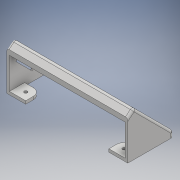
# Autodesk Inventor part: holder-LCD-screen
Saved by Autodesk Inventor 2018 (Build 220112000, 112)
## iProperties
Created: 2017-11-05
Part Number: holder-LCD-screen
Material: Generic
Document SubType Name: Modeling
Designer: Jurjen
Density: 1 g/cm^3
Appearance: Default
Author: Jurjen
Autodesk Inventor part; units mm, degrees
ref_plane "YZ Plane" through (0, 0, 0) normal (1, 0, 0) x (0, 1, 0)
ref_plane "XZ Plane" through (0, 0, 0) normal (0, 1, 0) x (-1, 0, 0)
ref_plane "XY Plane" through (0, 0, 0) normal (0, 0, 1) x (1, 0, 0)
sketch "Sketch1" plane through (0, 0, 0) normal (1, 0, 0) x (0, 1, 0)
  line L0 (-30, 25.7931) -> (-30, -25.7931)
  line L1 (30, -18.7931) -> (-21.6188, 32.8257)
  line L2 (-21.6188, 32.8257) -> (-30, 25.7931)
  line L3 (30, -18.7931) -> (30, -25.7931)
  line L4 (30, -25.7931) -> (-30, -25.7931)
  point P0 (0, 0)
  point P1 (-30, 0)
  point P2 (0, -25.7931)
  point P3 (-30, 0)
  dimension "d3" = 50
  dimension "d4" = 73
  dimension "d8" = 60
  dimension "d9" = 45
  dimension "d10" = 7
  constraints: 10 end point, 3 midpoint, 2 horizontal alignment, 2 vertical, 1 perpendicular, 1 vertical alignment
  measures "d3" angle of L2 L0
  measures "d4" distance of L1.start L1.end
  measures "d8" distance of L3.end L0.end
  measures "d9" angle of L4 L1
  measures "d10" distance of L1.start L3.end
extrude "Extrusion1" add sketch "Sketch1" along normal mid plane 160
sketch "Sketch2" plane through (-80, -21.6188, 32.8257) normal (0, 0.7071068, 0.7071068) x (1, 0, 0)
  line L0 (3.5, 69.5) -> (156.5, 69.5)
  line L1 (156.5, 69.5) -> (156.5, 3.5)
  line L2 (156.5, 3.5) -> (3.5, 3.5)
  line L3 (3.5, 3.5) -> (3.5, 69.5)
  line L4 (0, 0) -> (0, 73) projected
  line L5 (0, 0) -> (160, 0) projected
  line L6 (0, 73) -> (160, 73) projected
  line L7 (160, 73) -> (160, 0) projected
  point P0 (80, 38.4981)
  dimension "d11" = 3.5
  dimension "d12" = 3.5
  dimension "d13" = 3.5
  dimension "d14" = 3.5
  constraints: 8 end point, 2 parallel, 1 horizontal, 1 perpendicular
  measures "d11" distance between parallel lines of L4 L3
  measures "d12" distance between parallel lines of L5 L2
  measures "d13" distance between parallel lines of L6 L0
  measures "d14" distance between parallel lines of L7 L1
extrude "Extrusion2" cut sketch "Sketch2" against normal up to next contours L0 L1 L2 L3
sketch "Sketch3" plane through (-80, -21.6188, 32.8257) normal (0, 0.7071068, 0.7071068) x (1, 0, 0)
  line L0 (3.5, 3.5) -> (3.5, 69.5) projected
  line L1 (3.5, 69.5) -> (156.5, 69.5) projected
  line L2 (156.5, 69.5) -> (156.5, 3.5) projected
  line L3 (156.5, 3.5) -> (3.5, 3.5) projected
  line L4 (0, 0) -> (160, 0) projected
  line L5 (160, 73) -> (160, 0) projected
  line L6 (0, 73) -> (160, 73) projected
  line L7 (0, 0) -> (0, 73) projected
  line L8 (3.5, 69.5) -> (156.5, 69.5)
  line L9 (156.5, 69.5) -> (156.5, 3.5)
  line L10 (156.5, 3.5) -> (3.5, 3.5)
  line L11 (3.5, 3.5) -> (3.5, 69.5)
  line L12 (17.2, 55) -> (116.2, 55)
  line L13 (116.2, 55) -> (116.2, 14.5)
  line L14 (116.2, 14.5) -> (17.2, 14.5)
  line L15 (17.2, 14.5) -> (17.2, 55)
  circle A0 centre (142.6, 38.45) radius 2.75
  arc A1 (143.6, 56.45) -> (141.6, 56.45) centre (142.6, 56.45) ccw
  arc A2 (141.6, 52.45) -> (143.6, 52.45) centre (142.6, 52.45) ccw
  arc A3 (140.6, 54.95) -> (138.6, 54.95) centre (139.6, 54.95) ccw
  line L16 (141.6, 52.45) -> (141.6, 56.45)
  line L17 (143.6, 56.45) -> (143.6, 52.45)
  arc A4 (138.6, 53.95) -> (140.6, 53.95) centre (139.6, 53.95) ccw
  line L18 (138.6, 53.95) -> (138.6, 54.95)
  line L19 (140.6, 54.95) -> (140.6, 53.95)
  line L20 (142.6, 52.45) -> (142.6, 56.45) construction
  arc A5 (146.6, 54.95) -> (144.6, 54.95) centre (145.6, 54.95) ccw
  arc A6 (144.6, 53.95) -> (146.6, 53.95) centre (145.6, 53.95) ccw
  line L21 (146.6, 53.95) -> (146.6, 54.95)
  line L22 (144.6, 54.95) -> (144.6, 53.95)
  point P0 (80, 38.4981)
  dimension "d17" = 99
  dimension "d18" = 40.5
  dimension "d19" = 26.4
  dimension "d20" = 5.5
  dimension "d21" = 23.95
  dimension "d22" = 13.7
  dimension "d23" = 11
  dimension "d24" = 2
  dimension "d25" = 4
  dimension "d26" = 3
  dimension "d27" = 1.5
  dimension "d28" = 1.5
  dimension "d29" = 14
  constraints: 30 end point, 14 point on circle, 7 centre point, 7 symmetric about line, 6 tangent, 5 parallel, 3 equal radius, 3 vertical alignment, 2 horizontal, 2 perpendicular, 2 point on line, 2 vertical, 2 other
  measures "d17" distance between parallel lines of L13 L15
  measures "d18" distance between parallel lines of L14 L12
  measures "d19" distance from line of L13 A0.centre
  measures "d20" diameter of A0
  measures "d21" distance from line of A0.centre L14
  measures "d22" distance between parallel lines of L0 L15
  measures "d23" distance between parallel lines of L3 L14
  measures "d24" diameter of A1
  measures "d25" distance of L17.end L17.start
  measures "d26" horizontal distance of L20.end A3.centre
  measures "d27" vertical distance of L20.end A3.centre
  measures "d28" vertical distance of A4.centre L20.start
  measures "d29" distance of A0.centre L20.start
extrude "Extrusion3" add sketch "Sketch3" against normal blind 3 contours L0 L1 L2 L3
fillet "Fillet1" radius 3 8 edges at (0, -21.6188, 32.8257) (-80, 4.1906, 7.0163) (-80, -25.8094, 29.3094) (80, -25.8094, 29.3094) (80, 4.1906, 7.0163) (0, 30, -18.7931) (-80, 30, -22.2931) (80, 30, -22.2931)
sketch "Sketch4" plane through (76.5, 18.0503, -25.7931) normal (0, 0, -1) x (-1, 0, 0)
  line L0 (139.3, -2.8995) -> (139.3, -31.5373) projected
  line L1 (139.3, -31.5373) -> (40.3, -31.5373) projected
  line L2 (40.3, -31.5373) -> (40.3, -2.8995) projected
  line L3 (40.3, -2.8995) -> (139.3, -2.8995) projected
  ellipse E0 centre (13.9, -14.6021) end of major axis (16.65, -14.6021) minor radius 1.9445 projected
  line L4 (12.9, -4.7026) -> (12.9, -1.8742) projected
  ellipse E1 centre (13.9, -1.8742) end of major axis (12.9, -1.8742) minor radius 0.7071 (14.9, -1.8742) -> (12.9, -1.8742) ccw projected
  line L5 (14.9, -1.8742) -> (14.9, -4.7026) projected
  ellipse E2 centre (13.9, -4.7026) end of major axis (14.9, -4.7026) minor radius 0.7071 (12.9, -4.7026) -> (14.9, -4.7026) ccw projected
  ellipse E3 centre (10.9, -3.642) end of major axis (11.9, -3.642) minor radius 0.7071 (9.9, -3.642) -> (11.9, -3.642) ccw projected
  line L6 (9.9, -3.642) -> (9.9, -2.9349) projected
  ellipse E4 centre (10.9, -2.9349) end of major axis (9.9, -2.9349) minor radius 0.7071 (11.9, -2.9349) -> (9.9, -2.9349) ccw projected
  line L7 (11.9, -2.9349) -> (11.9, -3.642) projected
  ellipse E5 centre (16.9, -3.642) end of major axis (17.9, -3.642) minor radius 0.7071 (15.9, -3.642) -> (17.9, -3.642) ccw projected
  line L8 (15.9, -3.642) -> (15.9, -2.9349) projected
  ellipse E6 centre (16.9, -2.9349) end of major axis (15.9, -2.9349) minor radius 0.7071 (17.9, -2.9349) -> (15.9, -2.9349) ccw projected
  line L9 (17.9, -2.9349) -> (17.9, -3.642) projected
  line L10 (153, 7.3536) -> (153, -39.3155) projected
  line L11 (0, 7.3536) -> (153, 7.3536) projected
  line L12 (0, -39.3155) -> (0, 7.3536) projected
  line L13 (153, -39.3155) -> (0, -39.3155) projected
  line L14 (153, 0) -> (153, -48.0503) projected
  line L15 (0, 7.3536) -> (153, 7.3536)
  line L16 (153, 7.3536) -> (153, 0)
  line L17 (153, 0) -> (0, 0)
  line L18 (0, 0) -> (0, 7.3536)
  point P0 (76.5, -18.0503)
  constraints: 8 end point, 2 parallel, 1 horizontal, 1 perpendicular, 7 other
extrude "Extrusion4" cut sketch "Sketch4" against normal up to next contours L10 L17 L12 L11
sketch "Sketch5" plane through (-80, 0, 0) normal (-1, 0, 0) x (0, 0, 1)
  line L0 (-13.3123, -0.2295) -> (7.9009, -21.4427)
  line L1 (7.9009, -21.4427) -> (12.1436, -17.2001)
  line L2 (12.1436, -17.2001) -> (-9.0696, 4.0131)
  line L3 (-9.0696, 4.0131) -> (-13.3123, -0.2295)
  line L4 (-20.0357, 27) -> (28.7606, -21.7963) projected
  line L5 (28.2295, -21.2652) -> (-18.4395, 25.4038) projected
  line L6 (-18.4395, 25.4038) -> (28.2295, -21.2652) projected
  line L7 (-7.444, 14.4083) -> (-7.444, 14.4083) projected
  line L8 (-7.444, 14.4083) -> (-8.1511, 15.1154) projected
  line L9 (-8.1511, 15.1154) -> (-8.1511, 15.1154) projected
  line L10 (-8.1511, 15.1154) -> (-7.444, 14.4083) projected
  line L11 (-7.444, 14.4083) -> (-7.444, 14.4083) projected
  line L12 (-7.444, 14.4083) -> (-8.1511, 15.1154) projected
  line L13 (-8.1511, 15.1154) -> (-8.1511, 15.1154) projected
  line L14 (-8.1511, 15.1154) -> (-7.444, 14.4083) projected
  line L15 (-6.3833, 13.3476) -> (-9.2118, 16.1761) projected
  line L16 (-9.2118, 16.1761) -> (-9.2118, 16.1761) projected
  line L17 (-9.2118, 16.1761) -> (-6.3833, 13.3476) projected
  line L18 (-6.3833, 13.3476) -> (-6.3833, 13.3476) projected
  line L19 (5.4607, 1.5036) -> (1.5716, 5.3927) projected
  line L20 (-8.1865, 15.1508) -> (20.4514, -13.4871) projected
  line L21 (20.4514, -13.4871) -> (-8.1865, 15.1508) projected
  point P0 (0, 0)
  dimension "d35" = 30
  dimension "d36" = 6
  dimension "d39" = 14.5
  dimension "d40" = 15
  constraints: 8 end point, 3 perpendicular, 1 parallel
  measures "d35" distance of L1.end L2.end
  measures "d36" distance between parallel lines of L2 L0
  measures "d39" distance between parallel lines of L4 L0
  measures "d40" distance from line of L4.end L1
extrude "Extrusion5" cut sketch "Sketch5" against normal up to next
sketch "Sketch6" plane through (-77, -19.675, 30.8819) normal (0, 0.7071068, 0.7071068) x (1, 0, 0)
  circle A0 centre (4.1, 61.451) radius 1.6
  circle A1 centre (4.1, 11.951) radius 1.6
  circle A2 centre (148.6, 61.451) radius 1.6
  circle A3 centre (148.6, 11.951) radius 1.6
  line L0 (0.5, 71.9508) -> (0.5, 32.7743) projected
  line L1 (0.5, 0.751) -> (153.5, 0.751) projected
  point P0 (77, 35.7491)
  dimension "d41" = 3.2
  dimension "d42" = 144.5
  dimension "d43" = 49.5
  dimension "d44" = 3.6
  dimension "d45" = 11.2
  constraints: 4 centre point, 3 equal radius, 2 horizontal alignment, 2 vertical alignment
  measures "d41" diameter of A0
  measures "d42" distance of A2.centre A0.centre
  measures "d43" distance of A0.centre A1.centre
  measures "d44" distance from line of A0.centre L0
  measures "d45" distance from line of A1.centre L1
extrude "Extrusion6" cut sketch "Sketch6" against normal up to next
chamfer "Chamfer1" distance 2 angle 45 4 edges at (-80, -10.8361, -2.7057) (-80, 1.8918, -11.191) (-80, -6.5935, 1.537) (-80, -19.3214, 10.0222)
sketch "Sketch7" plane through (77, 30, -25.7931) normal (0, 0, -1) x (-1, 0, 0)
  line L0 (157, -51.7963) -> (157, -60) projected
  line L1 (157, -60) -> (132, -60)
  line L2 (132, -60) -> (132, -40)
  line L3 (132, -40) -> (157, -40)
  line L4 (157, -40) -> (157, -60)
  point P0 (77, -30)
  dimension "d51" = 25
  dimension "d52" = 20
  constraints: 8 end point, 2 parallel, 1 horizontal, 1 perpendicular
  measures "d51" distance between parallel lines of L4 L2
  measures "d52" distance between parallel lines of L1 L3
extrude "Extrusion7" add sketch "Sketch7" against normal blind 4
sketch "Sketch8" plane through (77, 30, -25.7931) normal (0, 0, -1) x (-1, 0, 0)
  circle A0 centre (142, -50) radius 2.1
  line L0 (157, -60) -> (132, -60) projected
  line L1 (132, -60) -> (132, -40) projected
  point P0 (77, -30)
  dimension "d55" = 10
  dimension "d56" = 10
  dimension "d57" = 4.2
  constraints: 1 centre point
  measures "d55" distance from line of L0 A0.centre
  measures "d56" distance from line of L1 A0.centre
  measures "d57" diameter of A0
fillet "Fillet2" radius 10 1 edges at (-55, -10, -23.7931)
extrude "Extrusion8" cut sketch "Sketch8" against normal up to next
mirror "Mirror1" about plane through (0, 0, 0) normal (1, 0, 0) of "Extrusion7", "Fillet2", "Extrusion8"
sketch "Sketch9" plane through (-77, -19.675, 30.8819) normal (0, 0.7071068, 0.7071068) x (1, 0, 0)
  line L0 (14.2, 64.6999) -> (52.5715, 64.6999) construction
  line L1 (52.5715, 64.6999) -> (52.5715, 56.5594) construction
  line L2 (52.5715, 56.5594) -> (14.2, 56.5594) construction
  line L3 (14.2, 56.5594) -> (14.2, 64.6999) construction
  line L4 (14.2, 52.251) -> (113.2, 52.251) projected
  line L5 (0, 69.0084) -> (154, 69.0084) projected
  line L6 (113.2, 52.251) -> (113.2, 69.0084) construction
  line L7 (20.0476, 60.6463) -> (18.5354, 60.3719)
  spline S0 degree 2 poles (18.5354, 60.3719) (18.4622, 60.8231) (17.9195, 61.2804) (17.4866, 61.2804) knots 0 0 0 1 2 2 2
  spline S1 degree 2 poles (17.4866, 61.2804) (16.9195, 61.2804) (16.2366, 60.4877) (16.2366, 59.5609) knots 0 0 0 1 2 2 2
  spline S2 degree 2 poles (16.2366, 59.5609) (16.2366, 58.5304) (16.9317, 57.6829) (17.511, 57.6829) knots 0 0 0 1 2 2 2
  spline S3 degree 2 poles (17.511, 57.6829) (17.95, 57.6829) (18.5049, 58.1829) (18.6207, 58.7865) knots 0 0 0 1 2 2 2
  line L8 (18.6207, 58.7865) -> (20.1268, 58.5304)
  spline S4 degree 2 poles (20.1268, 58.5304) (19.8951, 57.4938) (18.5598, 56.4329) (17.4439, 56.4329) knots 0 0 0 1 2 2 2
  spline S5 degree 2 poles (17.4439, 56.4329) (16.1756, 56.4329) (14.6634, 58.0365) (14.6634, 59.4572) knots 0 0 0 1 2 2 2
  spline S6 degree 2 poles (14.6634, 59.4572) (14.6634, 60.8902) (16.1756, 62.4877) (17.4683, 62.4877) knots 0 0 0 1 2 2 2
  spline S7 degree 2 poles (17.4683, 62.4877) (18.5293, 62.4877) (19.7732, 61.5792) (20.0476, 60.6463) knots 0 0 0 1 2 2 2
  spline S8 degree 2 poles (20.8585, 59.5426) (20.8585, 60.3048) (21.6146, 61.7377) (22.9927, 62.4877) (23.8463, 62.4877) knots 0 0 0 1 2 3 3 3
  spline S9 degree 2 poles (23.8463, 62.4877) (25.1634, 62.4877) (26.8463, 60.7804) (26.8463, 59.4755) knots 0 0 0 1 2 2 2
  spline S10 degree 2 poles (26.8463, 59.4755) (26.8463, 58.1646) (25.1451, 56.4329) (23.8585, 56.4329) knots 0 0 0 1 2 2 2
  spline S11 degree 2 poles (23.8585, 56.4329) (23.0598, 56.4329) (21.6146, 57.1524) (20.8585, 58.5426) (20.8585, 59.5426) knots 0 0 0 1 2 3 3 3
  spline S12 degree 2 poles (22.4317, 59.4633) (22.4317, 58.5975) (23.2488, 57.6829) (23.8524, 57.6829) knots 0 0 0 1 2 2 2
  spline S13 degree 2 poles (23.8524, 57.6829) (24.4561, 57.6829) (25.2671, 58.5975) (25.2671, 59.4694) knots 0 0 0 1 2 2 2
  spline S14 degree 2 poles (25.2671, 59.4694) (25.2671, 60.3231) (24.4561, 61.2377) (23.8524, 61.2377) knots 0 0 0 1 2 2 2
  spline S15 degree 2 poles (23.8524, 61.2377) (23.2488, 61.2377) (22.4317, 60.3231) (22.4317, 59.4633) knots 0 0 0 1 2 2 2
  line L9 (29.5171, 56.5609) -> (27.9805, 56.5609)
  line L10 (27.9805, 56.5609) -> (27.9805, 62.3597)
  line L11 (27.9805, 62.3597) -> (29.4073, 62.3597)
  line L12 (29.4073, 62.3597) -> (29.4073, 61.5365)
  spline S16 degree 2 poles (29.4073, 61.5365) (29.7732, 62.1219) (30.3524, 62.4877) (30.7244, 62.4877) knots 0 0 0 1 2 2 2
  spline S17 degree 2 poles (30.7244, 62.4877) (31.2488, 62.4877) (31.7305, 62.1951) knots 0 0 0 1 1 1
  line L13 (31.7305, 62.1951) -> (31.261, 60.8597)
  spline S18 degree 2 poles (31.261, 60.8597) (30.8707, 61.1097) (30.5415, 61.1097) knots 0 0 0 1 1 1
  spline S19 degree 2 poles (30.5415, 61.1097) (30.2183, 61.1097) (29.7732, 60.756) (29.5171, 59.8292) (29.5171, 58.3475) knots 0 0 0 1 2 3 3 3
  line L14 (29.5171, 58.3475) -> (29.5171, 56.5609)
  line L15 (35.7488, 58.4085) -> (37.2793, 58.1524)
  spline S20 degree 2 poles (37.2793, 58.1524) (36.9866, 57.3109) (35.7122, 56.4329) (34.7549, 56.4329) knots 0 0 0 1 2 2 2
  spline S21 degree 2 poles (34.7549, 56.4329) (33.2427, 56.4329) (32.5171, 57.4207) knots 0 0 0 1 1 1
  spline S22 degree 2 poles (32.5171, 57.4207) (31.9439, 58.2133) (31.9439, 59.4146) knots 0 0 0 1 1 1
  spline S23 degree 2 poles (31.9439, 59.4146) (31.9439, 60.8597) (33.45, 62.4877) (34.6024, 62.4877) knots 0 0 0 1 2 2 2
  spline S24 degree 2 poles (34.6024, 62.4877) (35.8951, 62.4877) (37.389, 60.7804) (37.3585, 59.0182) knots 0 0 0 1 2 2 2
  line L16 (37.3585, 59.0182) -> (33.5171, 59.0182)
  spline S25 degree 2 poles (33.5171, 59.0182) (33.5354, 58.3353) (34.2427, 57.5792) (34.7732, 57.5792) knots 0 0 0 1 2 2 2
  spline S26 degree 2 poles (34.7732, 57.5792) (35.1329, 57.5792) (35.6207, 57.9694) (35.7488, 58.4085) knots 0 0 0 1 2 2 2
  spline S27 degree 2 poles (35.8341, 59.9572) (35.8159, 60.6219) (35.1634, 61.317) (34.6939, 61.317) knots 0 0 0 1 2 2 2
  spline S28 degree 2 poles (34.6939, 61.317) (34.1939, 61.317) (33.8646, 60.9511) knots 0 0 0 1 1 1
  spline S29 degree 2 poles (33.8646, 60.9511) (33.5415, 60.5853) (33.5415, 59.9572) knots 0 0 0 1 1 1
  line L17 (33.5415, 59.9572) -> (35.8341, 59.9572)
  line L18 (40.758, 60.8592) -> (38.3018, 64.6999)
  line L19 (38.3018, 64.6999) -> (39.669, 64.6999)
  line L20 (39.669, 64.6999) -> (41.4184, 61.8382)
  line L21 (41.4184, 61.8382) -> (43.1679, 64.6999)
  line L22 (43.1679, 64.6999) -> (44.5408, 64.6999)
  line L23 (44.5408, 64.6999) -> (42.0846, 60.8592)
  line L24 (42.0846, 60.8592) -> (44.7667, 56.6999)
  line L25 (44.7667, 56.6999) -> (43.3996, 56.6999)
  line L26 (43.3996, 56.6999) -> (41.4184, 59.8802)
  line L27 (41.4184, 59.8802) -> (39.4431, 56.6999)
  line L28 (39.4431, 56.6999) -> (38.0759, 56.6999)
  line L29 (38.0759, 56.6999) -> (40.758, 60.8592)
  line L30 (45.039, 64.6999) -> (46.3134, 64.6999)
  line L31 (46.3134, 64.6999) -> (48.4742, 61.1547)
  line L32 (48.4742, 61.1547) -> (50.6291, 64.6999)
  line L33 (50.6291, 64.6999) -> (51.9094, 64.6999)
  line L34 (51.9094, 64.6999) -> (49.1346, 60.2336)
  line L35 (49.1346, 60.2336) -> (49.1346, 56.6999)
  line L36 (49.1346, 56.6999) -> (47.8543, 56.6999)
  line L37 (47.8543, 56.6999) -> (47.8543, 60.2336)
  line L38 (47.8543, 60.2336) -> (45.039, 64.6999)
  point P0 (77, 35.7491)
  point P1 (113.2, 60.6297)
  point P2 (14.2, 60.6297)
  constraints: 2 end point, 2 midpoint, 1 horizontal alignment, 1 point on line, 1 vertical, 1 vertical alignment, 2 other
emboss "Emboss1" sketch "Sketch9" operation cut depth 1 direction (0, -0.7071068, -0.7071068)
equation "\"d12\" = d11"
equation "\"d13\" = d11"
equation "\"d14\" = d11"
equation "\"d28\" = d27"
body "Solid1"
